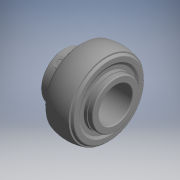
# Autodesk Inventor part: YAR 204-2LPW/SS-28.02014 -bearing
Saved by Autodesk Inventor 2017.3 (Build 213256000, 256)
## iProperties
Part Number: YAR 204-2LPW/SS-28.02014 -bearing
Material: Generic
Catalog Web Link: www.cadenas.de
Description: ayf_001hc_hh_hy_bearing-Y-bearings
Vendor: SKF
Document SubType Name: Modeling
Designer: partserver
Manufacturer: SKF
Mass: 16.4713 g
Surface Area: 186.321 cm^2
Volume: 16.4713 cm^3
Density: 1 g/cm^3
Appearance: PSOLRGB-175-175-175
Category: PARTsolutions
Company: SKF
Title: YAR 204-2LPW/SS-28.02014 -bearing
Author: Cadenas PARTsolutions
Comments: Y-bearings
PSOL_IDENT_0: {$CADENAS_DATA\23d-libs\skf\bearings_units_and_housings\bearing_units\ball_bearing_units\y-units\y-b
PSOL_IDENT_1: earing_square_flanged_units_parts\ayf_001hc_hh_hy_bearing.prj},225 {VTYP=3D},{NB=YAR 204-2LPW/SS-28.
PSOL_IDENT_2: 02014 -bearing},{LINA=YAR 204-2LPW/SS-28.02014 -bearing},{NN=ayf_001hc_hh_hy_bearing},{DATE=20.08.20
PSOL_IDENT_3: 20 13:45:20},{GEOMDATE=29.07.2020 17:09:33},{VERSION=},{LINEID=3320},{WBVAR=},{WBNUMERIC=}  {NB=YAR
PSOL_IDENT_4: 204-2LPW/SS-28.02014 -bearing},{LINA=YAR 204-2LPW/SS-28.02014 -bearing},{KT=DUMMY},{PRODUCTID=0},{DE
PSOL_IDENT_5: SIGNATION=YAR 204-2LPW/SS},{DD=20.0000},{D=47},{B=31.000},{C=14.000},{PITCH=33.500},{DW=7.938},{FO=I
PSOL_IDENT_6: EC_BBY_006},{DESIGN=ybrg1},{B1=MIN},{LM=Grub screw},{DES=Inner ring extended on both sides},{PS=},{M
PSOL_IDENT_7: AT=Stainless steel},{SS=},{UNIT=Inch},{G=MIN},{DD1=28.02},{DD2=MIN},{DD3=MIN},{B3=8.128},{B4=MIN},{B
PSOL_IDENT_8: B4=4.5},{R12=0.6},{R12X=0},{SS1=18.288},{NOTE=},{DG=MIN},{E=MIN},{F=MIN},{RG=MIN},{LOAD1=MIN},{LOAD2=
PSOL_IDENT_9: MIN},{LOAD3=MIN},{SPEED2=},{FF0=MIN},{BF=},{A15=},{A8=},{A4=},{BETA=},{SBT1=},{SBT2=},{RF1=},{RF2=},
PSOL_IDENT_10: {SF1=},{SF2=},{KZ=},{II=1},{Z=8},{SG=},{MASS=MIN},{G2=},{HEX=3.000},{RTT=},{MKIT=},{AS=},{TANGLE=},{
PSOL_IDENT_11: SLEEVE=},{SRING=},{FPC=},{POPI=},{NOUN=},{NOUNDES=},{MOD=},{MODDES=},{YZ=14.01},{PIM=YAR 204-2LPW-SS
PSOL_IDENT_12: },{LNDD11=MIN},{LUB3=1},{BZ=0.404133},{SDALG=h},{YRZ=20.719},{SHAPE=4},{LNB1HM11=0},{LWM=0},{TYPEID=
PSOL_IDENT_13: 0},{LUBGR2=0},{LOCKNUT=},{LOCKDEVICE=},{LNB=MIN},{BB=MIN},{LNB1=MIN},{S1ALG=18.288},{HH=MIN},{LDB=MI
PSOL_IDENT_14: N},{LDDD1=MIN},{LDDD2=MIN},{LDM=MIN},{LDFF=MIN},{TP=4},{LNBHM11=0},{BBHM11=0},{LNDD1HM11=0},{HELP=5}
PSOL_IDENT_15: ,{HHHM11=0},{LUBGR1=0},{LWV=0},{S2=23.4},{LUB2=0},{BZ1=0.000},{HEX2=}
NB: YAR 204-2LPW/SS-28.02014 -bearing
NN: ayf_001hc_hh_hy_bearing
NT: Y-bearings
NBSYN: $DESIGNATION.-$DD1.$PRODUCTID.$C.$B1.-bearing
LINA: YAR 204-2LPW/SS-28.02014 -bearing
CATALOG: SKF
DESIGNATION: YAR 204-2LPW/SS
DD: 20
D: 47
B: 31
C: 14
B1: 0
MAT: Stainless steel
DD1: 28.02
LOAD1: 0
LOAD2: 0
LOAD3: 0
SUPPLIER: SKF
ARTICLENO: YAR 204-2LPW/SS-28.02014 -bearing
BOMINFO: YAR 204-2LPW/SS-28.02014 -bearing
CREATOR: CADENAS GmbH
Autodesk Inventor part; units mm, degrees
ref_plane "YZ Plane" through (0, 0, 0) normal (1, 0, 0) x (0, 1, 0)
ref_plane "XZ Plane" through (0, 0, 0) normal (0, 1, 0) x (-1, 0, 0)
ref_plane "XY Plane" through (0, 0, 0) normal (0, 0, 1) x (1, 0, 0)
sketch "Sketch_1" plane through (0, 0, 0) normal (0, 0, 1) x (1, 0, 0)
  line L0 (50, 0) -> (-50, 0)
  arc A0 (-12.712, 10.6) -> (-12.112, 10) centre (-12.112, 10.6) ccw
  line L1 (-12.112, 10) -> (17.688, 10)
  arc A1 (17.688, 10) -> (18.288, 10.6) centre (17.688, 10.6) ccw
  line L2 (18.288, 10.6) -> (18.288, 13.41)
  arc A2 (18.288, 13.41) -> (17.688, 14.01) centre (17.688, 13.41) ccw
  line L3 (17.688, 14.01) -> (2.8715, 14.01)
  arc A3 (-2.8715, 14.01) -> (2.8715, 14.01) centre (0, 16.75) ccw
  line L4 (-2.8715, 14.01) -> (-12.112, 14.01)
  arc A4 (-12.112, 14.01) -> (-12.712, 13.41) centre (-12.112, 13.41) ccw
  line L5 (-12.712, 13.41) -> (-12.712, 10.6)
  constraints: 12 end point, 10 point on circle, 5 centre point
revolve "Revolution1" add sketch "Sketch_1" angle 360 about axis through (50, 0, 0) along (1, 0, 0)
sketch "Sketch_2" plane through (0, 10, 0) normal (0, 1, 0) x (1, 0, 0)
  circle A0 centre (13.788, 0) radius 3
  line L0 (12.288, -0.866) -> (13.788, -1.7321)
  line L1 (13.788, -1.7321) -> (15.288, -0.866)
  line L2 (15.288, -0.866) -> (15.288, 0.866)
  line L3 (15.288, 0.866) -> (13.788, 1.7321)
  line L4 (13.788, 1.7321) -> (12.288, 0.866)
  line L5 (12.288, 0.866) -> (12.288, -0.866)
  constraints: 12 end point, 1 centre point
extrude "Extrusion1" add sketch "Sketch_2" along normal blind 4.411
sketch "Sketch_3" plane through (0, -5, -8.6603) normal (0, -0.5, -0.8660254) x (1, 0, 0)
  circle A0 centre (13.788, 0) radius 3
  line L0 (12.288, -0.866) -> (13.788, -1.7321)
  line L1 (13.788, -1.7321) -> (15.288, -0.866)
  line L2 (15.288, -0.866) -> (15.288, 0.866)
  line L3 (15.288, 0.866) -> (13.788, 1.7321)
  line L4 (13.788, 1.7321) -> (12.288, 0.866)
  line L5 (12.288, 0.866) -> (12.288, -0.866)
  constraints: 12 end point, 1 centre point
extrude "Extrusion2" add sketch "Sketch_3" along normal blind 4.411
sketch "Sketch_16" plane through (0, 0, 0) normal (0, 0, 1) x (1, 0, 0)
  line L0 (7, 0) -> (-7, 0)
  line L1 (-7, 20.5419) -> (-5.0617, 20.5419)
  line L2 (-5.0617, 20.5419) -> (-4.9132, 20.6612)
  arc A0 (-4.5639, 20.5321) -> (-4.9132, 20.6612) centre (-4.7773, 20.4919) ccw
  line L3 (-4.5639, 20.5321) -> (-4.4804, 20.0882)
  arc A1 (-4.4804, 20.0882) -> (-4.2839, 19.9252) centre (-4.2839, 20.1252) ccw
  line L4 (-4.2839, 19.9252) -> (-2.4646, 19.9252)
  arc A2 (-2.4646, 19.9252) -> (-2.3164, 19.9729) centre (-2.4646, 20.1792) ccw
  arc A3 (2.3164, 19.9729) -> (-2.3164, 19.9729) centre (0, 16.75) ccw
  arc A4 (2.3164, 19.9729) -> (2.4646, 19.9252) centre (2.4646, 20.1792) ccw
  line L5 (2.4646, 19.9252) -> (4.2839, 19.9252)
  arc A5 (4.2839, 19.9252) -> (4.4804, 20.0882) centre (4.2839, 20.1252) ccw
  line L6 (4.4804, 20.0882) -> (4.5639, 20.5321)
  arc A6 (4.9132, 20.6612) -> (4.5639, 20.5321) centre (4.7773, 20.4919) ccw
  line L7 (4.9132, 20.6612) -> (5.0617, 20.5419)
  line L8 (5.0617, 20.5419) -> (7, 20.5419)
  line L9 (7, 20.5419) -> (7, 22.2856)
  arc A7 (7, 22.2856) -> (6.8584, 22.4769) centre (6.8, 22.2856) ccw
  arc A8 (6.8584, 22.4769) -> (-6.8584, 22.4769) centre (0, 0) ccw
  arc A9 (-6.8584, 22.4769) -> (-7, 22.2856) centre (-6.8, 22.2856) ccw
  line L10 (-7, 22.2856) -> (-7, 20.5419)
  constraints: 22 end point, 20 point on circle, 10 centre point
sketch "Sketch_30" plane through (0, 0, 0) normal (0, 0, 1) x (1, 0, 0)
  line L0 (7, 0) -> (-7, 0)
  line L1 (-7.8083, 20.2419) -> (-7, 19.7753)
  line L2 (-7, 19.7753) -> (-7, 18.7345)
  line L3 (-7, 18.7345) -> (-7.6062, 19.0845)
  line L4 (-7.6062, 19.0845) -> (-7.8083, 18.7345)
  line L5 (-7.8083, 18.7345) -> (-6.7874, 18.1451)
  line L6 (-6.7874, 18.1451) -> (-6.4967, 17.3394)
  line L7 (-6.4967, 17.3394) -> (-7.2562, 17.7779)
  line L8 (-7.2562, 17.7779) -> (-7.4583, 17.4279)
  line L9 (-7.4583, 17.4279) -> (-6.2841, 16.75)
  line L10 (-6.2841, 16.75) -> (-6.2841, 14.4141)
  line L11 (-6.2841, 14.4141) -> (-7.0924, 14.4141)
  line L12 (-7.0924, 14.4141) -> (-7.0924, 14.01)
  line L13 (-7.0924, 14.01) -> (-5.88, 14.01)
  line L14 (-5.88, 14.01) -> (-5.88, 16.75)
  line L15 (-5.88, 16.75) -> (-6.5959, 18.7345)
  line L16 (-6.5959, 18.7345) -> (-6.5959, 19.9878)
  arc A0 (-6.4459, 20.1378) -> (-6.5959, 19.9878) centre (-6.4459, 19.9878) ccw
  line L17 (-6.4459, 20.1378) -> (-4.5902, 20.1378)
  line L18 (-4.5902, 20.1378) -> (-4.5902, 20.5419)
  line L19 (-4.5902, 20.5419) -> (-6.7, 20.5419)
  arc A1 (-6.7, 20.5419) -> (-7, 20.2419) centre (-6.7, 20.2419) ccw
  line L20 (-7, 20.2419) -> (-7.6062, 20.5919)
  line L21 (-7.6062, 20.5919) -> (-7.8083, 20.2419)
  constraints: 44 end point, 4 point on circle, 2 centre point
revolve "Revolution2" add sketch "Sketch_30" angle 360 about axis through (7, 0, 0) along (1, 0, 0)
sketch "Sketch_31" plane through (0, 0, 0) normal (0, 0, 1) x (1, 0, 0)
  line L0 (7, 0) -> (-7, 0)
  line L1 (4.5902, 20.1378) -> (6.4459, 20.1378)
  arc A0 (6.5959, 19.9878) -> (6.4459, 20.1378) centre (6.4459, 19.9878) ccw
  line L2 (6.5959, 19.9878) -> (6.5959, 18.7345)
  line L3 (6.5959, 18.7345) -> (5.88, 16.75)
  line L4 (5.88, 16.75) -> (5.88, 14.01)
  line L5 (5.88, 14.01) -> (7.0924, 14.01)
  line L6 (7.0924, 14.01) -> (7.0924, 14.4141)
  line L7 (7.0924, 14.4141) -> (6.2841, 14.4141)
  line L8 (6.2841, 14.4141) -> (6.2841, 16.75)
  line L9 (6.2841, 16.75) -> (7.4583, 17.4279)
  line L10 (7.4583, 17.4279) -> (7.2562, 17.7779)
  line L11 (7.2562, 17.7779) -> (6.4967, 17.3394)
  line L12 (6.4967, 17.3394) -> (6.7874, 18.1451)
  line L13 (6.7874, 18.1451) -> (7.8083, 18.7345)
  line L14 (7.8083, 18.7345) -> (7.6062, 19.0845)
  line L15 (7.6062, 19.0845) -> (7, 18.7345)
  line L16 (7, 18.7345) -> (7, 19.7753)
  line L17 (7, 19.7753) -> (7.8083, 20.2419)
  line L18 (7.8083, 20.2419) -> (7.6062, 20.5919)
  line L19 (7.6062, 20.5919) -> (7, 20.2419)
  arc A1 (7, 20.2419) -> (6.7, 20.5419) centre (6.7, 20.2419) ccw
  line L20 (6.7, 20.5419) -> (4.5902, 20.5419)
  line L21 (4.5902, 20.5419) -> (4.5902, 20.1378)
  constraints: 44 end point, 4 point on circle, 2 centre point
revolve "Revolution3" add sketch "Sketch_31" angle 360 about axis through (7, 0, 0) along (1, 0, 0)
revolve "Revolution4" add sketch "Sketch_16" angle 360 about axis through (7, 0, 0) along (1, 0, 0)
sketch "Sketch_32" plane through (0, 0, 0) normal (0, 0, 1) x (1, 0, 0)
  line L0 (7, 0) -> (-7, 0)
  line L1 (7.2, 21.6785) -> (7.2, 21.4894)
  arc A0 (7.2, 21.4894) -> (7.2536, 21.3745) centre (7.35, 21.4894) ccw
  line L2 (7.2536, 21.3745) -> (7.9865, 20.7595)
  arc A1 (8.2008, 20.2998) -> (7.9865, 20.7595) centre (7.6008, 20.2998) ccw
  line L3 (8.2008, 20.2998) -> (8.2008, 19.473)
  line L4 (8.2008, 19.473) -> (7.7029, 19.7604)
  line L5 (7.7029, 19.7604) -> (7.5008, 19.4104)
  line L6 (7.5008, 19.4104) -> (8.2008, 19.0063)
  line L7 (8.2008, 19.0063) -> (8.2008, 18.073)
  line L8 (8.2008, 18.073) -> (7.5708, 18.4367)
  line L9 (7.5708, 18.4367) -> (7.3688, 18.0867)
  line L10 (7.3688, 18.0867) -> (8.0084, 17.7174)
  line L11 (8.0084, 17.7174) -> (7.485, 16.75)
  line L12 (7.485, 16.75) -> (7.485, 14.31)
  arc A2 (7.485, 14.31) -> (7.785, 14.01) centre (7.785, 14.31) ccw
  line L13 (7.785, 14.01) -> (9.8174, 14.01)
  line L14 (9.8174, 14.01) -> (9.8174, 14.4141)
  line L15 (9.8174, 14.4141) -> (8.0391, 14.4141)
  arc A3 (7.8891, 14.5641) -> (8.0391, 14.4141) centre (8.0391, 14.5641) ccw
  line L16 (7.8891, 14.5641) -> (7.8891, 16.75)
  line L17 (7.8891, 16.75) -> (8.605, 18.073)
  line L18 (8.605, 18.073) -> (8.605, 20.6248)
  arc A4 (8.605, 20.6248) -> (8.305, 21.1445) centre (8.005, 20.6248) ccw
  line L19 (8.305, 21.1445) -> (7.29, 21.7304)
  arc A5 (7.29, 21.7304) -> (7.2, 21.6785) centre (7.26, 21.6785) ccw
  constraints: 40 end point, 12 point on circle, 6 centre point
revolve "Revolution5" add sketch "Sketch_32" angle 360 about axis through (7, 0, 0) along (1, 0, 0)
sketch "Sketch_34" plane through (0, 0, 0) normal (0, 0, 1) x (1, 0, 0)
  line L0 (7, 0) -> (-7, 0)
  line L1 (-9.8174, 14.4141) -> (-9.8174, 14.01)
  line L2 (-9.8174, 14.01) -> (-7.785, 14.01)
  arc A0 (-7.785, 14.01) -> (-7.485, 14.31) centre (-7.785, 14.31) ccw
  line L3 (-7.485, 14.31) -> (-7.485, 16.75)
  line L4 (-7.485, 16.75) -> (-8.0084, 17.7174)
  line L5 (-8.0084, 17.7174) -> (-7.3688, 18.0867)
  line L6 (-7.3688, 18.0867) -> (-7.5708, 18.4367)
  line L7 (-7.5708, 18.4367) -> (-8.2008, 18.073)
  line L8 (-8.2008, 18.073) -> (-8.2008, 19.0063)
  line L9 (-8.2008, 19.0063) -> (-7.5008, 19.4104)
  line L10 (-7.5008, 19.4104) -> (-7.7029, 19.7604)
  line L11 (-7.7029, 19.7604) -> (-8.2008, 19.473)
  line L12 (-8.2008, 19.473) -> (-8.2008, 20.2998)
  arc A1 (-7.9865, 20.7595) -> (-8.2008, 20.2998) centre (-7.6008, 20.2998) ccw
  line L13 (-7.9865, 20.7595) -> (-7.2536, 21.3745)
  arc A2 (-7.2536, 21.3745) -> (-7.2, 21.4894) centre (-7.35, 21.4894) ccw
  line L14 (-7.2, 21.4894) -> (-7.2, 21.6785)
  arc A3 (-7.2, 21.6785) -> (-7.29, 21.7304) centre (-7.26, 21.6785) ccw
  line L15 (-7.29, 21.7304) -> (-8.305, 21.1445)
  arc A4 (-8.305, 21.1445) -> (-8.605, 20.6248) centre (-8.005, 20.6248) ccw
  line L16 (-8.605, 20.6248) -> (-8.605, 18.073)
  line L17 (-8.605, 18.073) -> (-7.8891, 16.75)
  line L18 (-7.8891, 16.75) -> (-7.8891, 14.5641)
  arc A5 (-8.0391, 14.4141) -> (-7.8891, 14.5641) centre (-8.0391, 14.5641) ccw
  line L19 (-8.0391, 14.4141) -> (-9.8174, 14.4141)
  constraints: 40 end point, 12 point on circle, 6 centre point
revolve "Revolution6" add sketch "Sketch_34" angle 360 about axis through (7, 0, 0) along (1, 0, 0)
ref_plane "ball_1_XY" through (0, 16.75, 0) normal (1, 0, 0) x (0, 0, -1)
ref_plane "ball_1_YZ" through (0, 16.75, 0) normal (0, 0, -1) x (0, 1, 0)
ref_plane "ball_1_ZX" through (0, 16.75, 0) normal (0, 1, 0) x (1, 0, 0)
ref_plane "ball_2_XY" through (0, 11.844, 11.844) normal (1, 0, 0) x (0, 0, -1)
ref_plane "ball_2_YZ" through (0, 11.844, 11.844) normal (0, 0, -1) x (0, 1, 0)
ref_plane "ball_2_ZX" through (0, 11.844, 11.844) normal (0, 1, 0) x (1, 0, 0)
ref_plane "ball_3_XY" through (0, 0, 16.75) normal (1, 0, 0) x (0, 0, -1)
ref_plane "ball_3_YZ" through (0, 0, 16.75) normal (0, 0, -1) x (0, 1, 0)
ref_plane "ball_3_ZX" through (0, 0, 16.75) normal (0, 1, 0) x (1, 0, 0)
ref_plane "ball_4_XY" through (0, -11.844, 11.844) normal (1, 0, 0) x (0, 0, -1)
ref_plane "ball_4_YZ" through (0, -11.844, 11.844) normal (0, 0, -1) x (0, 1, 0)
ref_plane "ball_4_ZX" through (0, -11.844, 11.844) normal (0, 1, 0) x (1, 0, 0)
ref_plane "ball_5_XY" through (0, -16.75, 0) normal (1, 0, 0) x (0, 0, -1)
ref_plane "ball_5_YZ" through (0, -16.75, 0) normal (0, 0, -1) x (0, 1, 0)
ref_plane "ball_5_ZX" through (0, -16.75, 0) normal (0, 1, 0) x (1, 0, 0)
ref_plane "ball_6_XY" through (0, -11.844, -11.844) normal (1, 0, 0) x (0, 0, -1)
ref_plane "ball_6_YZ" through (0, -11.844, -11.844) normal (0, 0, -1) x (0, 1, 0)
ref_plane "ball_6_ZX" through (0, -11.844, -11.844) normal (0, 1, 0) x (1, 0, 0)
ref_plane "ball_7_XY" through (0, 0, -16.75) normal (1, 0, 0) x (0, 0, -1)
ref_plane "ball_7_YZ" through (0, 0, -16.75) normal (0, 0, -1) x (0, 1, 0)
ref_plane "ball_7_ZX" through (0, 0, -16.75) normal (0, 1, 0) x (1, 0, 0)
ref_plane "ball_8_XY" through (0, 11.844, -11.844) normal (1, 0, 0) x (0, 0, -1)
ref_plane "ball_8_YZ" through (0, 11.844, -11.844) normal (0, 0, -1) x (0, 1, 0)
ref_plane "ball_8_ZX" through (0, 11.844, -11.844) normal (0, 1, 0) x (1, 0, 0)
ref_plane "brg_XY" through (0, 0, 0) normal (1, 0, 0) x (0, 0, -1)
ref_plane "brg_YZ" through (0, 0, 0) normal (0, 0, -1) x (0, 1, 0)
ref_plane "brg_ZX" through (0, 0, 0) normal (0, 1, 0) x (1, 0, 0)
ref_plane "brg3_XY" through (18.288, 0, 0) normal (1, 0, 0) x (0, 0, -1)
ref_plane "brg3_YZ" through (18.288, 0, 0) normal (0, 0, -1) x (0, 1, 0)
ref_plane "brg3_ZX" through (18.288, 0, 0) normal (0, 1, 0) x (1, 0, 0)
body "Solid1"
